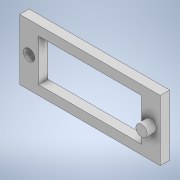
# Autodesk Inventor part: Eslabon_1_inventor
Saved by Autodesk Inventor 2021 (Build 250183000, 183)
## iProperties
Created: 2021-08-13
Part Number: Eslabon_1_inventor
Material: Genérico
Document SubType Name: Modeling
Designer: uriel
Density: 1 g/cm^3
Appearance: Valor por defecto
Author: uriel
Autodesk Inventor part; units mm, degrees
ref_plane "YZ Plane" through (0, 0, 0) normal (1, 0, 0) x (0, 1, 0)
ref_plane "XZ Plane" through (0, 0, 0) normal (0, 1, 0) x (-1, 0, 0)
ref_plane "XY Plane" through (0, 0, 0) normal (0, 0, 1) x (1, 0, 0)
sketch "Boceto1" plane through (0, 0, 0) normal (0, 0, 1) x (1, 0, 0)
  circle A0 centre (0, 0) radius 6
  line L0 (-10, -32.5) -> (10, -32.5)
  line L1 (10, -32.5) -> (10, 32.5)
  line L2 (10, 32.5) -> (-10, 32.5)
  line L3 (-10, 32.5) -> (-10, -32.5)
  line L4 (-10, -32.5) -> (10, 32.5) construction
  line L5 (10, -32.5) -> (-10, 32.5) construction
  line L6 (0, 0) -> (84.0619, 0)
  line L7 (0, 0) -> (130, 0)
  circle A1 centre (130, 0) radius 6
  line L8 (120, -32.5) -> (140, -32.5)
  line L9 (140, -32.5) -> (140, 32.5)
  line L10 (140, 32.5) -> (120, 32.5)
  line L11 (120, 32.5) -> (120, -32.5)
  line L12 (120, -32.5) -> (140, 32.5) construction
  line L13 (140, -32.5) -> (120, 32.5) construction
  line L14 (10, -32.5) -> (120, -32.5)
  line L15 (120, -32.5) -> (120, -22.5)
  line L16 (120, -22.5) -> (10, -22.5)
  line L17 (120, 32.5) -> (120, 22.5)
  line L18 (120, 22.5) -> (10, 22.5)
  line L19 (10, 32.5) -> (120, 32.5)
  dimension "d0" = 12
  dimension "d1" = 130
  dimension "d2" = 65
  dimension "d3" = 20
  dimension "d4" = 20
  dimension "d5" = 65
  dimension "d6" = 10
  dimension "d7" = 10
  constraints: 40 end point, 5 point on line, 4 midpoint, 4 parallel, 4 perpendicular, 3 horizontal, 2 centre point, 2 coincident
  measures "d0" diameter of A0
  measures "d1" distance of L6.start L7.end
  measures "d2" distance of L0.end L1.end
  measures "d3" distance of L1.end L2.end
  measures "d4" distance of L10.end L9.end
  measures "d5" distance of L8.end L9.end
  measures "d6" distance of L8.start L15.end
  measures "d7" distance of L10.end L17.end
extrude "Extrusión1" add sketch "Boceto1" along normal blind 10 contours L3 L2 L1 L0 | L1 L16 L11 L14 | L11 L10 L9 L8 | L19 L11 L18 L1 | A1
sketch "Boceto2" plane through (0, 0, 10) normal (0, 0, 1) x (1, 0, 0)
  circle A0 centre (0, 0) radius 6 projected
  line L0 (0, 0) -> (130, 0)
  circle A1 centre (130, 0) radius 6
  dimension "d10" = 130
  dimension "d11" = 12
  constraints: 2 end point, 1 centre point, 1 coincident, 1 horizontal
  measures "d10" distance of L0.start L0.end
  measures "d11" diameter of A1
extrude "Extrusión2" add sketch "Boceto2" along normal blind 10 contours A1
